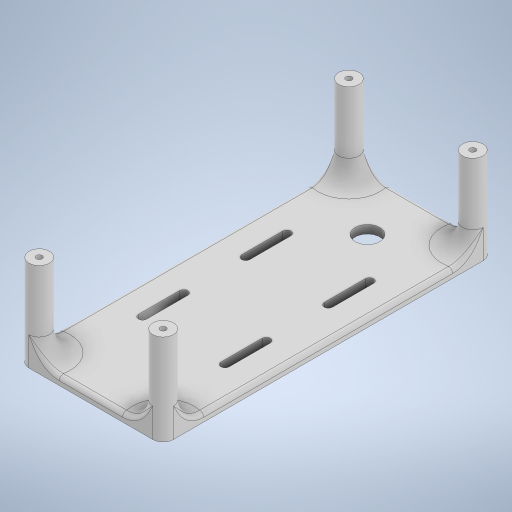
# Autodesk Inventor part: 2
Saved by Autodesk Inventor 2023 (Build 270158000, 158)
## iProperties
Created: 2025-03-08
Part Number: 2
Material: Generic
Document SubType Name: Modeling
Designer: micha
Density: 1 g/cm^3
Appearance: Default
Author: micha
Autodesk Inventor part; units mm, degrees
ref_plane "YZ Plane" through (0, 0, 0) normal (1, 0, 0) x (0, 1, 0)
ref_plane "XZ Plane" through (0, 0, 0) normal (0, 1, 0) x (-1, 0, 0)
ref_plane "XY Plane" through (0, 0, 0) normal (0, 0, 1) x (1, 0, 0)
sketch "Sketch1" plane through (0, 0, 0) normal (0, 1, 0) x (-1, 0, 0)
  line L0 (-30, 80) -> (30, 80)
  line L1 (35, 75) -> (35, -75)
  line L2 (30, -80) -> (-30, -80)
  line L3 (-35, -75) -> (-35, 75)
  line L4 (-35, 80) -> (35, -80) construction
  line L5 (35, 80) -> (-35, -80) construction
  arc A0 (35, 75) -> (30, 80) centre (30, 75) ccw
  arc A1 (-30, 80) -> (-35, 75) centre (-30, 75) ccw
  arc A2 (30, -80) -> (35, -75) centre (30, -75) ccw
  arc A3 (-35, -75) -> (-30, -80) centre (-30, -75) ccw
  point P0 (0, 0)
  dimension "d0" = 160
  dimension "d1" = 70
  dimension "d2" = 5
  dimension "d3" = 5
  dimension "d4" = 5
  constraints: 12 end point, 8 point on circle, 8 point on line, 8 tangent, 4 centre point, 2 midpoint, 2 parallel, 1 equal radius, 1 horizontal, 1 perpendicular
  measures "d0" distance between parallel lines of L2 L0
  measures "d1" distance between parallel lines of L3 L1
  measures "d2" radius of A0
  measures "d3" radius of A1
  measures "d4" radius of A2
extrude "Extrusion1" add sketch "Sketch1" along normal blind 4
sketch "Sketch2" plane through (0, 4, 0) normal (0, 1, 0) x (1, 0, 0)
  arc A0 (-35, -75) -> (-30, -80) centre (-30, -75) ccw projected
  circle A1 centre (-30, -75) radius 5
  point P0 (0, 0)
  point P1 (-30, -80)
  constraints: 1 coincident, 3 other
extrude "Extrusion2" add sketch "Sketch2" along normal blind 40
mirror "Mirror1" about plane through (0, 0, 0) normal (0, 0, 1) of "Extrusion2"
mirror "Mirror2" about plane through (0, 0, 0) normal (1, 0, 0) of "Extrusion2", "Mirror1"
fillet "Fillet1" radius 10 4 edges at (-26.4645, 4, 71.4645) (-26.4645, 4, -71.4645) (26.4645, 4, -71.4645) (26.4645, 4, 71.4645)
fillet "Fillet2" radius 2 12 edges at (35, 7.1699, -69.1496) (35, 7.1698, 69.1495) (35, 4, 0) (-35, 7.1699, 69.1496) (-35, 7.0477, -68.9976) (-35, 4, 0) (24.1495, 7.1698, 80) (-24.1496, 7.1699, 80) (0, 4, 80) (0, 4, -80) (24.1496, 7.1699, -80) (-24.1495, 7.1698, -80)
sketch "Sketch4" plane through (-30, 44, 75) normal (0, 1, 0) x (1, 0, 0)
  circle A0 centre (0, 0) radius 5 projected
  arc A1 (0, 155) -> (-5, 150) centre (0, 150) ccw projected
  arc A2 (65, 150) -> (60, 155) centre (60, 150) ccw projected
  circle A3 centre (60, 0) radius 5 projected
  point P0 (30, 75)
  constraints: 4 coincident
hole "Hole1" at (-30, 44, 75) at (-30, 44, -75) at (30, 44, -75) at (30, 44, 75) direction (0, -1, 0) diameter 2.9 depth 20 tip angle 118 clearance for "Flat Head Machine Screw" size "M2.5" standard "Ansi Metric M Profile"
sketch "Sketch6" plane through (0, 0, 0) normal (0, -1, 0) x (1, 0, 0)
  line L0 (20, 35) -> (20, 15) construction
  line L1 (18, 35) -> (18, 15)
  line L2 (22, 15) -> (22, 35)
  arc A0 (22, 35) -> (18, 35) centre (20, 35) ccw
  arc A1 (18, 15) -> (22, 15) centre (20, 15) ccw
  point P0 (0, 0)
  point P1 (20, 25)
  dimension "d27" = 4
  dimension "d28" = 20
  dimension "d29" = 20
  dimension "d31" = 25
  constraints: 8 end point, 4 point on circle, 4 tangent, 2 centre point, 1 midpoint, 1 parallel, 1 vertical
  measures "d27" distance between parallel lines of L1 L2
  measures "d28" distance of L0.start L0.end
  measures "d29" horizontal distance of point (20, 25) point (0, 0)
  measures "d31" vertical distance of point (20, 25) point (0, 0)
extrude "Extrusion3" cut sketch "Sketch6" against normal blind 10
mirror "Mirror3" about plane through (0, 0, 0) normal (0, 0, 1) of "Extrusion3"
mirror "Mirror4" about plane through (0, 0, 0) normal (1, 0, 0) of "Extrusion3", "Mirror3"
sketch "Sketch7" plane through (0, 0, 0) normal (0, -1, 0) x (1, 0, 0)
  circle A0 centre (0, -54) radius 6
  point P0 (0, 0)
  dimension "d34" = 12
  dimension "d35" = 54
  constraints: 1 centre point, 1 vertical alignment
  measures "d34" diameter of A0
  measures "d35" distance of point (0, 0) A0.centre
extrude "Extrusion4" cut sketch "Sketch7" against normal blind 10
body "Solid1"
